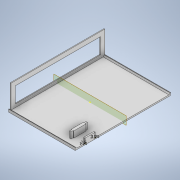
# Autodesk Inventor part: lower casing
Saved by Autodesk Inventor 2020 (Build 240168000, 168)
## iProperties
Created: 2019-06-23
Part Number: lower casing
Material: Generic
Document SubType Name: Modeling
Designer: jjsch
Density: 1 g/cm^3
Appearance: Default
Mass: 57.7992 g
Surface Area: 519.548 cm^2
Volume: 57.7992 cm^3
Author: jjsch
Autodesk Inventor part; units mm, degrees
ref_plane "YZ Plane" through (0, 0, 0) normal (1, 0, 0) x (0, 1, 0)
ref_plane "XZ Plane" through (0, 0, 0) normal (0, 1, 0) x (-1, 0, 0)
ref_plane "XY Plane" through (0, 0, 0) normal (0, 0, 1) x (1, 0, 0)
sketch "Sketch1" plane through (0, 0, 0) normal (0, 1, 0) x (-1, 0, 0)
  line L0 (-60, -84) -> (60, -84)
  line L1 (60, -84) -> (60, 84)
  line L2 (60, 84) -> (-60, 84)
  line L3 (-60, 84) -> (-60, -84)
  line L4 (-60, -84) -> (60, 84) construction
  line L5 (60, -84) -> (-60, 84) construction
  point P0 (0, 0)
  dimension "d0" = 168
  dimension "d1" = 120
  constraints: 12 end point, 2 midpoint, 2 parallel, 1 horizontal, 1 perpendicular
  measures "d0" distance of L1.end L0.end
  measures "d1" distance of L1.end L2.end
extrude "Extrusion1" add sketch "Sketch1" along normal blind 2.4
sketch "Sketch2" plane through (0, 2.4, 0) normal (0, 1, 0) x (1, 0, 0)
  line L0 (60, -84) -> (60, 84) projected
  line L1 (60, -68.75) -> (57.6, -68.75)
  line L2 (57.6, -68.75) -> (57.6, -51.25)
  line L3 (57.6, -51.25) -> (60, -51.25)
  line L4 (60, -51.25) -> (60, -68.75)
  line L5 (-60, -84) -> (60, -84) projected
  point P0 (0, 0)
  dimension "d4" = 2.4
  dimension "d5" = 17.5
  dimension "d6" = 15.25
  constraints: 8 end point, 2 parallel, 1 horizontal, 1 perpendicular, 1 point on line
  measures "d4" distance of L2.end L3.end
  measures "d5" distance of L1.end L2.end
  measures "d6" distance between parallel lines of L5 L1
extrude "Extrusion2" add sketch "Sketch2" along normal blind 8.25
sketch "Sketch3" plane through (0, 2.4, 0) normal (0, 1, 0) x (1, 0, 0)
  line L0 (59.425, -52.5) -> (58.175, -52.5)
  line L1 (58.175, -52.5) -> (58.175, -50)
  line L2 (58.175, -50) -> (59.425, -50)
  line L3 (59.425, -50) -> (59.425, -52.5)
  line L4 (57.6, -51.25) -> (60, -51.25) projected
  line L5 (59.425, -52.5) -> (58.175, -50) construction
  line L6 (58.175, -52.5) -> (59.425, -50) construction
  line L7 (59.425, -67.5) -> (58.175, -67.5)
  line L8 (58.175, -67.5) -> (58.175, -70)
  line L9 (58.175, -70) -> (59.425, -70)
  line L10 (59.425, -70) -> (59.425, -67.5)
  line L11 (60, -68.75) -> (57.6, -68.75) projected
  line L12 (59.425, -67.5) -> (58.175, -70) construction
  line L13 (58.175, -67.5) -> (59.425, -70) construction
  point P0 (0, 0)
  point P1 (58.8, -51.25)
  point P2 (58.8, -68.75)
  point P3 (59.425, -68.75)
  point P4 (58.175, -68.75)
  point P5 (58.175, -51.25)
  point P6 (59.425, -51.25)
  dimension "d9" = 1.25
  dimension "d10" = 2.5
  dimension "d11" = 1.25
  dimension "d12" = 2.5
  constraints: 24 end point, 6 midpoint, 4 parallel, 2 horizontal, 2 perpendicular
  measures "d9" distance of L1.end L2.end
  measures "d10" distance of L0.end L1.end
  measures "d11" distance of L9.end L8.end
  measures "d12" distance of L8.end L7.end
extrude "Extrusion3" add sketch "Sketch3" along normal blind 8.25 contours L4 L1 L2 L3 | L10 L9 L8 L11
sketch "Sketch4" plane through (0, 2.4, 0) normal (0, 1, 0) x (1, 0, 0)
  line L0 (60, -84) -> (60, -68.75) projected
  line L1 (-60, -84) -> (60, -84) projected
  line L2 (41.5, -71) -> (36.5, -71)
  line L3 (36.5, -71) -> (36.5, -49)
  line L4 (36.5, -49) -> (41.5, -49)
  line L5 (41.5, -49) -> (41.5, -71)
  line L6 (40.3125, -67) -> (37.6875, -67)
  line L7 (37.6875, -67) -> (37.6875, -75)
  line L8 (37.6875, -75) -> (40.3125, -75)
  line L9 (40.3125, -75) -> (40.3125, -67)
  line L10 (40.3125, -67) -> (37.6875, -75) construction
  line L11 (37.6875, -67) -> (40.3125, -75) construction
  line L12 (40.3125, -53) -> (37.6875, -53)
  line L13 (37.6875, -53) -> (37.6875, -45)
  line L14 (37.6875, -45) -> (40.3125, -45)
  line L15 (40.3125, -45) -> (40.3125, -53)
  line L16 (40.3125, -53) -> (37.6875, -45) construction
  line L17 (37.6875, -53) -> (40.3125, -45) construction
  point P0 (0, 0)
  point P1 (39, -71)
  point P2 (39, -49)
  point P3 (40.3125, -71)
  point P4 (37.6875, -71)
  point P5 (37.6875, -49)
  point P6 (40.3125, -49)
  dimension "d15" = 18.5
  dimension "d16" = 13
  dimension "d17" = 5
  dimension "d18" = 22
  dimension "d21" = 2.625
  dimension "d22" = 8
  dimension "d23" = 2.625
  dimension "d24" = 8
  constraints: 32 end point, 6 midpoint, 6 parallel, 3 horizontal, 3 perpendicular
  measures "d15" distance from line of L0 L2.start
  measures "d16" distance from line of L1 L2.start
  measures "d17" distance of L3.end L4.end
  measures "d18" distance of L2.end L3.end
  measures "d21" distance of L8.end L7.end
  measures "d22" distance of L7.end L6.end
  measures "d23" distance of L13.end L14.end
  measures "d24" distance of L12.end L13.end
extrude "Extrusion4" add sketch "Sketch4" along normal blind 11.25
sketch "Sketch5" plane through (0, 2.4, 0) normal (0, 1, 0) x (1, 0, 0)
  point P0 (0, 0)
sketch "Sketch6" plane through (60, 0, 84) normal (1, 0, 0) x (0, 0, -1)
  line L0 (0, 0) -> (168, 0) projected
  line L1 (0, 0) -> (-3, 0)
  line L2 (-3, 0) -> (-3, 4.7)
  line L3 (-3, 4.7) -> (0, 4.7)
  line L4 (0, 4.7) -> (0, 0)
  line L5 (0, 4.7) -> (3, 4.7) construction
  line L6 (-3, 4.7) -> (0, 4.7) construction
  line L7 (-2.1213, 4.5213) -> (0, 2.4)
  line L8 (-2.1213, 4.5213) -> (-2.0713, 4.5213)
  line L9 (0, 2.4) -> (15.25, 2.4) projected
  line L10 (-0.4669, 0) -> (0, 0)
  line L11 (0, 0) -> (0, 2.4) projected
  line L12 (-0.4669, 0) -> (0, 0)
  line L13 (-0.4669, 0) -> (0, 0)
  line L14 (-2.0713, 4.5213) -> (-2.0713, 4.7)
  line L15 (0, 0) -> (-3, 3)
  line L16 (0, 0) -> (4.2426, 0) construction
  point P0 (84, 0)
  point P1 (-3, 2.4)
  point P2 (-2.5884, 2.4)
  point P3 (0, 2.4)
  point P4 (-2.0713, 4.7)
  dimension "d25" = 3
  dimension "d26" = 4.7
  dimension "d31" = 3
  dimension "d33" = 0
  dimension "d39" = 45
  dimension "d44" = 2.4
  dimension "d45" = 2.4
  dimension "d46" = 135
  constraints: 28 end point, 7 horizontal, 4 point on line, 2 parallel, 2 perpendicular, 1 collinear, 1 equal length
  measures "d25" distance of L2.end L3.end
  measures "d26" distance of L1.end L2.end
  measures "d31" distance of L7.start L7.end
  measures "d33" distance from line of L4 L7.end
  measures "d39" angle of L8 L7
  measures "d44" distance of L0.start L7.end
  measures "d45" distance between parallel lines of L0 L9
  measures "d46" angle of L16 L15
extrude "Extrusion5" add sketch "Sketch6" against normal up to surface (120 mm away) contours L15 L2 L3 L14 L8 L7 L4 | L1 L2 L15
ref_plane "Work Plane2" through (0, 2.4, 0) normal (0, 0, -1) x (-1, 0, 0)
mirror "Mirror2" about plane through (0, 2.4, 0) normal (0, 0, -1) of "Extrusion5"
sketch "Sketch7" plane through (-60, 0, 87) normal (-1, 0, 0) x (0, 0, 1)
  line L0 (-174, 0) -> (0, 0) projected
  line L1 (0, 4.7) -> (0, 0) projected
  line L2 (-0.9287, 4.7) -> (0, 4.7) projected
  line L3 (-0.9287, 4.5213) -> (-0.9287, 4.7) projected
  line L4 (-0.8787, 4.5213) -> (-0.9287, 4.5213) projected
  line L5 (-3, 2.4) -> (-0.8787, 4.5213) projected
  line L6 (-171, 2.4) -> (-3, 2.4) projected
  line L7 (-171, 2.4) -> (-173.1213, 4.5213) projected
  line L8 (-173.1213, 4.5213) -> (-173.0713, 4.5213) projected
  line L9 (-173.0713, 4.5213) -> (-173.0713, 4.7) projected
  line L10 (-173.0713, 4.7) -> (-174, 4.7) projected
  line L11 (-174, 4.7) -> (-174, 0) projected
  line L12 (-174, 4.7) -> (-174, 0) projected
  line L13 (-174, 0) -> (-2.972, 0)
  line L14 (-2.972, 0) -> (-2.972, 44.842)
  line L15 (-2.972, 44.842) -> (-174, 44.842)
  line L16 (-174, 44.842) -> (-174, 0)
  point P0 (-87, 0)
  point P1 (-2.972, 2.428)
  dimension "d47" = 171.028
  dimension "d48" = 44.842
  constraints: 8 end point, 2 parallel, 1 horizontal, 1 perpendicular
  measures "d47" distance of L15.end L14.end
  measures "d48" distance of L14.end L13.end
extrude "Extrusion6" add sketch "Sketch7" along normal blind 1.5
sketch "Sketch8" plane through (-61.5, 0, 87) normal (-1, 0, 0) x (0, 0, 1)
  line L0 (0, 0) -> (0, 4.7) projected
  line L1 (0, 4.7) -> (-0.9287, 4.7) projected
  line L2 (-0.9287, 4.7) -> (-0.9287, 4.5213) projected
  line L3 (-0.9287, 4.5213) -> (-0.8787, 4.5213) projected
  line L4 (-0.8787, 4.5213) -> (-2.972, 2.428) projected
  line L5 (-2.972, 2.428) -> (-2.972, 44.842) projected
  line L6 (-2.972, 44.842) -> (-174, 44.842) projected
  line L7 (-174, 44.842) -> (-174, 0) projected
  line L8 (-174, 0) -> (0, 0) projected
  line L9 (-166, 36.842) -> (-10.972, 36.842)
  line L10 (-10.972, 36.842) -> (-10.972, 8)
  line L11 (-10.972, 8) -> (-166, 8)
  line L12 (-166, 8) -> (-166, 36.842)
  point P0 (-87, 0)
  dimension "d51" = 8
  constraints: 8 end point, 3 other
  measures "d51" distance between parallel lines of L6 L9
extrude "Extrusion7" cut sketch "Sketch8" against normal blind 1.5 contours L9 L10 L11 L12
sketch "Sketch9" plane through (-61.5, 0, 87) normal (-1, 0, 0) x (0, 0, 1)
  point P0 (-87, 0)
body "Solid1"
